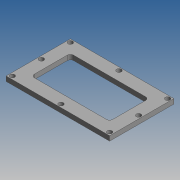
# Autodesk Inventor part: P021_HautEcranProtecLidar
Saved by Autodesk Inventor 2021.3 (Build 253353000, 353)
## iProperties
Created: 2021-11-12
Part Number: P021_HautEcranProtecLidar
Material: Générique
Document SubType Name: Modeling
Designer: gabri
Density: 1 g/cm^3
Appearance: Par défaut
Author: gabri
Autodesk Inventor part; units mm, degrees
ref_plane "YZ Plane" through (0, 0, 0) normal (1, 0, 0) x (0, 1, 0)
ref_plane "XZ Plane" through (0, 0, 0) normal (0, 1, 0) x (-1, 0, 0)
ref_plane "XY Plane" through (0, 0, 0) normal (0, 0, 1) x (1, 0, 0)
sketch "Sketch2" plane through (0, 0, 0) normal (0, 0, 1) x (1, 0, 0)
  line L0 (33, -20.5) -> (-33, -20.5)
  line L1 (-33, -20.5) -> (-33, 20.5)
  line L2 (-33, 20.5) -> (33, 20.5)
  line L3 (33, 20.5) -> (33, -20.5)
  line L4 (33, -20.5) -> (-33, 20.5) construction
  line L5 (-33, -20.5) -> (33, 20.5) construction
  line L6 (23, -12.5) -> (-23, -12.5)
  line L7 (-25, -10.5) -> (-25, 10.5)
  line L8 (-23, 12.5) -> (23, 12.5)
  line L9 (25, 10.5) -> (25, -10.5)
  line L10 (25, -12.5) -> (-25, 12.5) construction
  line L11 (-25, -12.5) -> (25, 12.5) construction
  arc A0 (-23, 12.5) -> (-25, 10.5) centre (-23, 10.5) ccw
  arc A1 (-25, -10.5) -> (-23, -12.5) centre (-23, -10.5) ccw
  arc A2 (23, -12.5) -> (25, -10.5) centre (23, -10.5) ccw
  arc A3 (25, 10.5) -> (23, 12.5) centre (23, 10.5) ccw
  point P0 (0, 0)
  dimension "d0" = 66
  dimension "d1" = 41
  dimension "d4" = 8
  dimension "d5" = 8
  dimension "d6" = 2
  constraints: 24 end point, 8 point on circle, 8 point on line, 8 tangent, 4 centre point, 4 midpoint, 4 parallel, 3 equal radius, 2 horizontal, 2 perpendicular
  measures "d0" distance of L1.end L2.end
  measures "d1" distance of L0.end L1.end
  measures "d4" distance between parallel lines of L2 L8
  measures "d5" distance between parallel lines of L1 L7
  measures "d6" radius of A0
extrude "Extrusion1" add sketch "Sketch2" along normal blind 3
sketch "Sketch3" plane through (0, 0, 3) normal (0, 0, 1) x (1, 0, 0)
  line L0 (-33, -20.5) -> (33, -20.5) construction
  line L1 (33, -20.5) -> (33, 20.5) construction
  line L2 (-33, 20.5) -> (-33, -20.5) construction
  line L3 (33, 20.5) -> (-33, 20.5) construction
  line L4 (-46.2, 0) -> (46.2, 0) construction
  line L5 (0, 28.7) -> (0, -28.7) construction
  point P0 (0, 0)
  point P1 (31, -18.5)
  point P2 (31, 0)
  point P3 (31, 18.5)
  point P4 (0, 18.5)
  point P5 (-31, 18.5)
  point P6 (-31, 0)
  point P7 (-31, -18.5)
  point P8 (0, -18.5)
  dimension "d7" = 2
  dimension "d8" = 2
  dimension "d9" = 2
  dimension "d10" = 2
  dimension "d11" = 2
  dimension "d12" = 2
  dimension "d13" = 2
  dimension "d14" = 2
  dimension "d15" = 2
  dimension "d16" = 2
  dimension "d17" = 2
  dimension "d18" = 2
  constraints: 4 point on line
  measures "d7" distance from line of L0 point (31, -18.5)
  measures "d8" distance from line of L1 point (31, -18.5)
  measures "d9" distance from line of L0 point (0, -18.5)
  measures "d10" distance from line of L0 point (-31, -18.5)
  measures "d11" distance from line of L2 point (-31, -18.5)
  measures "d12" distance from line of L2 point (-31, 0)
  measures "d13" distance from line of L2 point (-31, 18.5)
  measures "d14" distance from line of L3 point (-31, 18.5)
  measures "d15" distance from line of L3 point (0, 18.5)
  measures "d16" distance from line of L3 point (31, 18.5)
  measures "d17" distance from line of L1 point (31, 18.5)
  measures "d18" distance from line of L1 point (31, 0)
hole "Hole1" at (31, -18.5, 3) at (31, 0, 3) at (31, 18.5, 3) at (0, 18.5, 3) at (-31, 18.5, 3) at (-31, 0, 3) at (-31, -18.5, 3) at (0, -18.5, 3) direction (0, 0, -1) diameter 3 depth 8.8 tip angle 118
body "Solid1"
